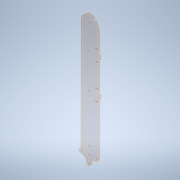
# Autodesk Inventor part: 関節2_側板
Saved by Autodesk Inventor 2021 (Build 250183000, 183)
## iProperties
Created: 2022-02-02
Part Number: 関節2_側板
Material: ポリカーボネート、スモーク
Document SubType Name: Modeling
Designer: hirohumi
Mass: 212.972 g
Surface Area: 311.279 cm^2
Volume: 78.8784 cm^3
Density: 1.2 g/cm^3
Appearance: ポリカーボネート - スモーク
Author: hirohumi
Autodesk Inventor part; units mm, degrees
ref_plane "YZ Plane" through (0, 0, 0) normal (1, 0, 0) x (0, 1, 0)
ref_plane "XZ Plane" through (0, 0, 0) normal (0, 1, 0) x (-1, 0, 0)
ref_plane "XY Plane" through (0, 0, 0) normal (0, 0, 1) x (1, 0, 0)
sketch "スケッチ1" plane through (0, 0, 0) normal (0, 0, 1) x (1, 0, 0)
  circle A0 centre (0, 0) radius 1.6
  circle A1 centre (0, 0) radius 20 construction
  circle A2 centre (0, 20) radius 1.6
  circle A3 centre (-20, 0) radius 1.6
  circle A4 centre (0, -20) radius 1.6
  circle A5 centre (20, 0) radius 1.6
  circle A6 centre (0, 300) radius 1.6
  arc A7 (18.7663, 306.9157) -> (-20, 300) centre (0, 300) ccw
  line L0 (-20, 300) -> (-20, 13.2288)
  arc A8 (-23.75, 3.3072) -> (-20, -5) centre (-20, 0) ccw
  arc A9 (-5, -20) -> (5, -20) centre (0, -20) ccw
  arc A10 (20, -5) -> (25, 0) centre (20, 0) ccw
  arc A11 (-23.75, 3.3072) -> (-20, 13.2288) centre (-35, 13.2288) ccw
  arc A12 (-5, -20) -> (-20, -5) centre (-20, -20) ccw
  arc A13 (20, -5) -> (5, -20) centre (20, -20) ccw
  line L1 (25, 240) -> (28, 240)
  line L2 (28, 240) -> (28, 230)
  line L3 (28, 230) -> (25, 230)
  arc A14 (25, 243) -> (25, 240) centre (25, 241.5) ccw
  arc A15 (25, 230) -> (25, 227) centre (25, 228.5) ccw
  line L4 (25, 150) -> (28, 150)
  line L5 (28, 150) -> (28, 140)
  line L6 (28, 140) -> (25, 140)
  arc A16 (25, 153) -> (25, 150) centre (25, 151.5) ccw
  arc A17 (25, 140) -> (25, 137) centre (25, 138.5) ccw
  line L7 (18.7663, 306.9157) -> (25, 290)
  line L8 (25, 290) -> (25, 250.5385)
  line L9 (25, 227) -> (25, 220.5385)
  line L10 (25, 137) -> (25, 130.5385)
  circle A18 centre (0, 235) radius 1.6
  circle A19 centre (0, 145) radius 1.6
  arc A20 (25, 250.5385) -> (25, 249.4615) centre (26.4, 250) ccw
  arc A21 (25, 220.5385) -> (25, 219.4615) centre (26.4, 220) ccw
  arc A22 (25, 160.5385) -> (25, 159.4615) centre (26.4, 160) ccw
  arc A23 (25, 130.5385) -> (25, 129.4615) centre (26.4, 130) ccw
  arc A24 (25, 249.4615) -> (25, 250.5385) centre (26.4, 250) ccw construction
  line L11 (25, 249.4615) -> (25, 243)
  line L12 (25, 250.5385) -> (25, 249.4615) construction
  arc A25 (25, 219.4615) -> (25, 220.5385) centre (26.4, 220) ccw construction
  line L13 (25, 220.5385) -> (25, 219.4615) construction
  line L14 (25, 219.4615) -> (25, 160.5385)
  line L15 (25, 159.4615) -> (25, 153)
  line L16 (25, 160.5385) -> (25, 159.4615) construction
  arc A26 (25, 159.4615) -> (25, 160.5385) centre (26.4, 160) ccw construction
  arc A27 (25, 129.4615) -> (25, 130.5385) centre (26.4, 130) ccw construction
  line L17 (25, 129.4615) -> (25, 0)
  line L18 (25, 130.5385) -> (25, 129.4615) construction
  point P0 (28, 235)
  dimension "d0" = 3.2
  dimension "d1" = 40
  dimension "d2" = 3.2
  dimension "d3" = 3.2
  dimension "d4" = 3.2
  dimension "d5" = 3.2
  dimension "d6" = 3.2
  dimension "d7" = 300
  dimension "d8" = 20
  dimension "d9" = 5
  dimension "d10" = 5
  dimension "d11" = 5
  dimension "d12" = 15
  dimension "d14" = 15
  dimension "d15" = 15
  dimension "d18" = 3
  dimension "d19" = 3
  dimension "d20" = 1.5
  dimension "d21" = 1.5
  dimension "d22" = 1.5
  dimension "d23" = 1.5
  dimension "d24" = 10
  dimension "d25" = 10
  dimension "d26" = 10
  dimension "d27" = 60
  dimension "d28" = 80
  dimension "d29" = 3.2
  dimension "d30" = 3.2
  dimension "d31" = 90
  dimension "d34" = 3
  dimension "d35" = 3
  dimension "d36" = 3
  dimension "d37" = 3
  dimension "d38" = 10
  dimension "d39" = 10
  dimension "d40" = 1.4
  dimension "d41" = 1.4
  dimension "d42" = 1.4
  dimension "d43" = 10
  dimension "d44" = 10
  dimension "d45" = 1.4
  constraints: 42 point on circle, 38 end point, 28 centre point, 15 tangent, 12 vertical, 9 vertical alignment, 6 coincident, 4 perpendicular, 3 horizontal alignment, 2 horizontal, 2 parallel, 1 midpoint, 1 point on line
  measures "d0" diameter of A0
  measures "d1" diameter of A1
  measures "d2" diameter of A2
  measures "d3" diameter of A3
  measures "d4" diameter of A4
  measures "d5" diameter of A5
  measures "d6" diameter of A6
  measures "d7" distance of point (0, 0) A6.centre
  measures "d8" radius of A7
  measures "d9" radius of A8
  measures "d10" radius of A9
  measures "d11" radius of A10
  measures "d12" radius of A11
  measures "d14" radius of A13
  measures "d15" radius of A12
  measures "d18" distance of L1.start L1.end
  measures "d19" distance of L4.start L4.end
  measures "d20" radius of A14
  measures "d21" radius of A15
  measures "d22" radius of A16
  measures "d23" radius of A17
  measures "d24" distance of L4.end L6.start
  measures "d25" distance of L1.end L2.end
  measures "d26" vertical distance of A6.centre L7.end
  measures "d27" distance from line of L1 A6.centre
  measures "d28" distance between parallel lines of L4 L3
  measures "d29" diameter of A18
  measures "d30" diameter of A19
  measures "d31" distance of A19.centre A18.centre
  measures "d34" diameter of A20
  measures "d35" diameter of A21
  measures "d36" diameter of A22
  measures "d37" diameter of A23
  measures "d38" distance from line of L4 A22.centre
  measures "d39" distance from line of A23.centre L6
  measures "d40" distance from line of L10 A23.centre
  measures "d41" distance from line of L9 A22.centre
  measures "d42" distance from line of L9 A21.centre
  measures "d43" distance from line of A21.centre L3
  measures "d44" distance from line of L1 A20.centre
  measures "d45" distance from line of L8 A20.centre
extrude "押し出し2" add sketch "スケッチ1" along normal blind 6
sketch "スケッチ2" plane through (25, 160.5385, 0) normal (1, 0, 0) x (0, 0, -1)
  circle A0 centre (-3, -0.5385) radius 1.25
  circle A1 centre (-3, -30.5385) radius 1.25
  circle A2 centre (-3, 59.4615) radius 1.25
  circle A3 centre (-3, 89.4615) radius 1.25
  line L0 (0, 82.4615) -> (0, 88.923) projected
  line L1 (0, 79.4615) -> (-6, 79.4615) projected
  line L2 (0, 69.4615) -> (-6, 69.4615) projected
  line L3 (0, -10.5385) -> (-6, -10.5385) projected
  line L4 (0, -20.5385) -> (-6, -20.5385) projected
  point P0 (0, -160.5385)
  dimension "d46" = 2.5
  dimension "d47" = 2.5
  dimension "d48" = 2.5
  dimension "d49" = 2.5
  dimension "d50" = 3
  dimension "d51" = 10
  dimension "d52" = 10
  dimension "d53" = 10
  dimension "d54" = 10
  constraints: 4 centre point, 3 vertical alignment
  measures "d46" diameter of A0
  measures "d47" diameter of A1
  measures "d48" diameter of A2
  measures "d49" diameter of A3
  measures "d50" distance from line of L0 A3.centre
  measures "d51" distance from line of A3.centre L1
  measures "d52" distance from line of A2.centre L2
  measures "d53" distance from line of L3 A0.centre
  measures "d54" distance from line of A1.centre L4
extrude "押し出し3" cut sketch "スケッチ2" against normal blind 10
